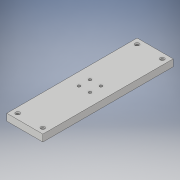
# Autodesk Inventor part: Grabber Platform
Saved by Autodesk Inventor 2019.4 (Build 234330000, 330)
## iProperties
Created: 2020-12-03
Part Number: Grabber Platform
Material: Generic
Document SubType Name: Modeling
Designer: caleb
Density: 1 g/cm^3
Appearance: Default
Author: caleb
Autodesk Inventor part; units mm, degrees
ref_plane "YZ Plane" through (0, 0, 0) normal (1, 0, 0) x (0, 1, 0)
ref_plane "XZ Plane" through (0, 0, 0) normal (0, 1, 0) x (-1, 0, 0)
ref_plane "XY Plane" through (0, 0, 0) normal (0, 0, 1) x (1, 0, 0)
sketch "Sketch1" plane through (0, 0, 0) normal (0, 1, 0) x (-1, 0, 0)
  line L0 (-13.15, 47.5) -> (13.15, 47.5)
  line L1 (13.15, 47.5) -> (13.15, -47.5)
  line L2 (13.15, -47.5) -> (-13.15, -47.5)
  line L3 (-13.15, -47.5) -> (-13.15, 47.5)
  line L4 (-13.15, 47.5) -> (13.15, -47.5) construction
  line L5 (13.15, 47.5) -> (-13.15, -47.5) construction
  point P0 (0, 0)
  dimension "d0" = 95
  dimension "d1" = 26.3
  constraints: 12 end point, 2 midpoint, 2 parallel, 1 horizontal, 1 perpendicular
  measures "d0" distance of L0.end L1.end
  measures "d1" distance of L0.start L0.end
extrude "Extrusion1" add sketch "Sketch1" along normal blind 5
sketch "Sketch2" plane through (0, 0, 0) normal (0, -1, 0) x (1, 0, 0)
  circle A0 centre (4, -4) radius 1.5
  circle A1 centre (4, 4) radius 1.5
  circle A2 centre (-4, 4) radius 1.5
  circle A3 centre (-4, -4) radius 1.5
  point P0 (0, 0)
  dimension "d4" = 3
  dimension "d5" = 4
  dimension "d6" = 4
  dimension "d7" = 4
  dimension "d8" = 4
  constraints: 4 centre point, 3 equal radius, 2 horizontal alignment, 2 vertical alignment
  measures "d4" diameter of A1
  measures "d5" horizontal distance of point (0, 0) A1.centre
  measures "d6" horizontal distance of A1.centre point (0, 0)
  measures "d7" horizontal distance of point (0, 0) A0.centre
  measures "d8" horizontal distance of point (0, 0) A3.centre
hole "Hole1" at (4, 0, 4) at (4, 0, -4) at (-4, 0, -4) at (-4, 0, 4) direction (0, 1, 0) diameter 2 end through all countersink diameter 3.0226 countersink angle 82
sketch "Sketch3" plane through (0, 5, 0) normal (0, 1, 0) x (1, 0, 0)
  circle A0 centre (-9.15, -43.5) radius 1.5
  circle A1 centre (9.15, -43.5) radius 1.5
  circle A2 centre (9.15, 43.5) radius 1.5
  circle A3 centre (-9.15, 43.5) radius 1.5
  line L0 (13.15, 47.5) -> (-13.15, 47.5) projected
  line L1 (13.15, -47.5) -> (13.15, 47.5) projected
  point P0 (0, 0)
  point P1 (-13.15, -47.5)
  dimension "d16" = 3
  dimension "d17" = 4
  dimension "d18" = 4
  dimension "d19" = 4
  dimension "d20" = 4
  constraints: 4 centre point, 3 equal radius, 2 horizontal alignment, 2 vertical alignment
  measures "d16" diameter of A0
  measures "d17" horizontal distance of A0.centre point (-13.15, -47.5)
  measures "d18" horizontal distance of A0.centre point (-13.15, -47.5)
  measures "d19" distance from line of L0 A3.centre
  measures "d20" distance from line of L1 A2.centre
hole "Hole2" at (-9.15, 5, 43.5) at (9.15, 5, 43.5) at (9.15, 5, -43.5) at (-9.15, 5, -43.5) direction (0, -1, 0) diameter 2 end through all countersink diameter 3.0226 countersink angle 82
body "Solid1"
